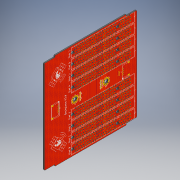
# Autodesk Inventor part: Backplane_PCB
Saved by Autodesk Inventor 2018 (Build 220112000, 112)
## iProperties
Created: 2018-10-18
Part Number: Backplane_PCB
Material: Epoxy Resin
Document SubType Name: Modeling
Designer: Bradley
Density: 1.14 g/cm^3
Appearance: Smooth - Dark Gray
Author: Bradley
Autodesk Inventor part; units mm, degrees
ref_plane "YZ Plane" through (0, 0, 0) normal (1, 0, 0) x (0, 1, 0)
ref_plane "XZ Plane" through (0, 0, 0) normal (0, 1, 0) x (-1, 0, 0)
ref_plane "XY Plane" through (0, 0, 0) normal (0, 0, 1) x (1, 0, 0)
sketch "Sketch11" plane through (0, 0, 0) normal (1, 0, 0) x (0, 1, 0)
  line L0 (-41.4, 41.6) -> (-32, 41.6)
  line L1 (-32, 41.6) -> (-32, 43)
  line L2 (-32, 43) -> (32, 43)
  line L3 (32, 43) -> (32, 41.6)
  line L4 (32, 41.6) -> (41.4, 41.6)
  line L5 (41.4, 41.6) -> (41.4, -41.6)
  line L6 (41.4, -41.6) -> (32, -41.6)
  line L7 (32, -41.6) -> (32, -43)
  line L8 (32, -43) -> (-32, -43)
  line L9 (-32, -43) -> (-32, -41.6)
  line L10 (-32, -41.6) -> (-41.4, -41.6)
  line L11 (-41.4, -41.6) -> (-41.4, 41.6)
  point P0 (0, 0)
  point P1 (0, 43)
  point P2 (-41.4, 0)
  dimension "d86" = 83.2
  dimension "d87" = 9.4
  dimension "d88" = 82.8
  dimension "d89" = 86
  constraints: 24 end point, 8 perpendicular, 5 point on line, 3 collinear, 2 midpoint, 1 horizontal, 1 horizontal alignment, 1 vertical, 1 vertical alignment
  measures "d86" distance of L4.end L5.end
  measures "d87" distance of L3.end L4.end
  measures "d88" distance between parallel lines of L11 L5
  measures "d89" distance between parallel lines of L8 L2
extrude "Extrusion3" add sketch "Sketch11" along normal mid plane 1
fillet "Fillet2" radius 0.5 12 edges at (0, -32, 43) (0, -32, 41.6) (0, -41.4, 41.6) (0, -32, -41.6) (0, -32, -43) (0, -41.4, -41.6) (0, 32, -43) (0, 32, -41.6) (0, 41.4, -41.6) (0, 32, 43) (0, 32, 41.6) (0, 41.4, 41.6)
sketch "Sketch12" plane through (0.5, 0, 0) normal (1, 0, 0) x (0, 0, -1)
  arc A0 (-41.1, 41.4) -> (-41.6, 40.9) centre (-41.1, 40.9) ccw projected
  line L0 (-41.6, 40.9) -> (-41.6, 32.5) projected
  arc A1 (-42.1, 32) -> (-41.6, 32.5) centre (-42.1, 32.5) ccw projected
  line L1 (-42.1, 32) -> (-42.5, 32) projected
  arc A2 (-42.5, 32) -> (-43, 31.5) centre (-42.5, 31.5) ccw projected
  line L2 (-43, 31.5) -> (-43, -31.5) projected
  arc A3 (-43, -31.5) -> (-42.5, -32) centre (-42.5, -31.5) ccw projected
  line L3 (-42.5, -32) -> (-42.1, -32) projected
  arc A4 (-41.6, -32.5) -> (-42.1, -32) centre (-42.1, -32.5) ccw projected
  line L4 (-41.6, -32.5) -> (-41.6, -40.9) projected
  arc A5 (-41.6, -40.9) -> (-41.1, -41.4) centre (-41.1, -40.9) ccw projected
  line L5 (-41.1, -41.4) -> (41.1, -41.4) projected
  arc A6 (41.1, -41.4) -> (41.6, -40.9) centre (41.1, -40.9) ccw projected
  line L6 (41.6, -40.9) -> (41.6, -32.5) projected
  arc A7 (42.1, -32) -> (41.6, -32.5) centre (42.1, -32.5) ccw projected
  line L7 (42.1, -32) -> (42.5, -32) projected
  arc A8 (42.5, -32) -> (43, -31.5) centre (42.5, -31.5) ccw projected
  line L8 (43, -31.5) -> (43, 31.5) projected
  arc A9 (43, 31.5) -> (42.5, 32) centre (42.5, 31.5) ccw projected
  line L9 (42.5, 32) -> (42.1, 32) projected
  arc A10 (41.6, 32.5) -> (42.1, 32) centre (42.1, 32.5) ccw projected
  line L10 (41.6, 32.5) -> (41.6, 40.9) projected
  arc A11 (41.6, 40.9) -> (41.1, 41.4) centre (41.1, 40.9) ccw projected
  line L11 (41.1, 41.4) -> (-41.1, 41.4) projected
  line L12 (-42.9956, -41.4) -> (-42.9956, 41.4) construction
  line L13 (-42.9956, 41.4) -> (42.9956, 41.4) construction
  line L14 (42.9956, 41.4) -> (42.9956, -41.4) construction
  line L15 (42.9956, -41.4) -> (-42.9956, -41.4) construction
  line L16 (-41.1, -41.4) -> (41.1, -41.4) projected
  point P0 (0, 0)
  point P1 (0, -41.4)
  point P2 (0, -41.4)
  constraints: 3 midpoint, 2 collinear, 2 other
decal "Decal3"
sketch "Sketch13" plane through (-0.5, 0, 0) normal (-1, 0, 0) x (0, 0, 1)
  arc A0 (41.6, 40.9) -> (41.1, 41.4) centre (41.1, 40.9) ccw projected
  line L0 (41.1, 41.4) -> (-41.1, 41.4) projected
  arc A1 (-41.1, 41.4) -> (-41.6, 40.9) centre (-41.1, 40.9) ccw projected
  line L1 (-41.6, 40.9) -> (-41.6, 32.5) projected
  arc A2 (-42.1, 32) -> (-41.6, 32.5) centre (-42.1, 32.5) ccw projected
  line L2 (-42.1, 32) -> (-42.5, 32) projected
  arc A3 (-42.5, 32) -> (-43, 31.5) centre (-42.5, 31.5) ccw projected
  line L3 (-43, 31.5) -> (-43, -31.5) projected
  arc A4 (-43, -31.5) -> (-42.5, -32) centre (-42.5, -31.5) ccw projected
  line L4 (-42.5, -32) -> (-42.1, -32) projected
  arc A5 (-41.6, -32.5) -> (-42.1, -32) centre (-42.1, -32.5) ccw projected
  line L5 (-41.6, -32.5) -> (-41.6, -40.9) projected
  arc A6 (-41.6, -40.9) -> (-41.1, -41.4) centre (-41.1, -40.9) ccw projected
  line L6 (-41.1, -41.4) -> (41.1, -41.4) projected
  arc A7 (41.1, -41.4) -> (41.6, -40.9) centre (41.1, -40.9) ccw projected
  line L7 (41.6, -40.9) -> (41.6, -32.5) projected
  arc A8 (42.1, -32) -> (41.6, -32.5) centre (42.1, -32.5) ccw projected
  line L8 (42.1, -32) -> (42.5, -32) projected
  arc A9 (42.5, -32) -> (43, -31.5) centre (42.5, -31.5) ccw projected
  line L9 (43, -31.5) -> (43, 31.5) projected
  arc A10 (43, 31.5) -> (42.5, 32) centre (42.5, 31.5) ccw projected
  line L10 (42.5, 32) -> (42.1, 32) projected
  arc A11 (41.6, 32.5) -> (42.1, 32) centre (42.1, 32.5) ccw projected
  line L11 (41.6, 32.5) -> (41.6, 40.9) projected
  line L12 (41.1, 41.4) -> (-41.1, 41.4) projected
  line L13 (42.9956, 41.4) -> (42.9956, -41.4) construction
  line L14 (42.9956, -41.4) -> (-42.9956, -41.4) construction
  line L15 (-42.9956, -41.4) -> (-42.9956, 41.4) construction
  line L16 (-42.9956, 41.4) -> (42.9956, 41.4) construction
  line L17 (-41.1, -41.4) -> (41.1, -41.4) projected
  point P0 (0, 0)
  point P1 (0, -41.4)
  point P2 (0, -41.4)
  constraints: 3 midpoint, 2 collinear, 2 other
decal "Decal4"
sketch "Sketch14" plane through (0.5, 0, 0) normal (1, 0, 0) x (0, 0, -1)
  point P0 (0, 0)
  point P1 (0, -14)
  point P2 (0, 14)
  constraints: 2 other
hole "Hole7" at (0.5, -14, 0) at (0.5, 14, 0) direction (-1, 0, 0) diameter 3.3 end through all
sketch "Sketch15" plane through (0.5, 0, 0) normal (1, 0, 0) x (0, 0, -1)
  point P0 (0, 0)
  point P1 (37.5, 24)
  point P2 (37.5, -16.15)
  point P3 (-37.5, 24)
  point P4 (-37.5, -16.15)
  point P5 (28.5, 24)
  point P6 (28.5, -16.15)
  point P7 (19.5, 24)
  point P8 (19.5, -16.15)
  point P9 (10.5, 24)
  point P10 (10.5, -16.15)
  point P11 (-10.5, 24)
  point P12 (-10.5, -16.15)
  point P13 (-19.5, 24)
  point P14 (-19.5, -16.15)
  point P15 (-28.5, 24)
  point P16 (-28.5, -16.15)
  constraints: 16 other
hole "Hole8" at (0.5, 24, -37.5) at (0.5, -16.15, -37.5) at (0.5, 24, 37.5) at (0.5, -16.15, 37.5) at (0.5, 24, -28.5) at (0.5, -16.15, -28.5) at (0.5, 24, -19.5) at (0.5, -16.15, -19.5) at (0.5, 24, -10.5) at (0.5, -16.15, -10.5) at (0.5, 24, 10.5) at (0.5, -16.15, 10.5) at (0.5, 24, 19.5) at (0.5, -16.15, 19.5) at (0.5, 24, 28.5) at (0.5, -16.15, 28.5) direction (-1, 0, 0) diameter 2.35 end through all
sketch "Sketch16" plane through (0.5, 0, 0) normal (1, 0, 0) x (0, 0, -1)
  point P0 (0, 0)
  point P1 (40.75, 0.65)
  point P2 (-29.75, -6.35)
  point P3 (-31.75, -7.35)
  point P4 (-25.25, -7.35)
  point P5 (-27.25, -8.35)
  point P6 (-29.75, -8.35)
  point P7 (-31.75, -9.35)
  point P8 (-25.25, -9.35)
  point P9 (-27.25, -10.35)
  point P10 (-29.75, -10.35)
  point P11 (-31.75, -11.35)
  point P12 (-25.25, -11.35)
  point P13 (-27.25, -12.35)
  point P14 (-29.75, -12.35)
  point P15 (-31.75, -13.35)
  point P16 (-25.25, -13.35)
  point P17 (-27.25, -14.35)
  point P18 (36.25, 25.65)
  point P19 (34.25, 26.65)
  point P20 (40.75, 26.65)
  point P21 (38.75, 25.65)
  point P22 (36.25, 27.65)
  point P23 (34.25, 28.65)
  point P24 (40.75, 28.65)
  point P25 (38.75, 27.65)
  point P26 (36.25, 29.65)
  point P27 (34.25, 30.65)
  point P28 (40.75, 30.65)
  point P29 (38.75, 29.65)
  point P30 (36.25, 31.65)
  point P31 (34.25, 32.65)
  point P32 (40.75, 32.65)
  point P33 (38.75, 31.65)
  point P34 (36.25, 33.65)
  point P35 (34.25, 34.65)
  point P36 (40.75, 34.65)
  point P37 (38.75, 33.65)
  point P38 (36.25, 35.65)
  point P39 (38.75, 35.65)
  point P40 (34.25, 22.65)
  point P41 (40.75, 22.65)
  point P42 (38.75, 21.65)
  point P43 (36.25, 21.65)
  point P44 (34.25, 20.65)
  point P45 (40.75, 20.65)
  point P46 (38.75, 19.65)
  point P47 (36.25, 19.65)
  point P48 (34.25, 18.65)
  point P49 (40.75, 18.65)
  point P50 (38.75, 17.65)
  point P51 (36.25, 17.65)
  point P52 (34.25, 16.65)
  point P53 (40.75, 16.65)
  point P54 (38.75, 15.65)
  point P55 (36.25, 15.65)
  point P56 (34.25, 14.65)
  point P57 (40.75, 14.65)
  point P58 (38.75, 13.65)
  point P59 (36.25, 13.65)
  point P60 (34.25, 12.65)
  point P61 (40.75, 12.65)
  point P62 (38.75, 11.65)
  point P63 (36.25, 11.65)
  point P64 (34.25, 10.65)
  point P65 (40.75, 10.65)
  point P66 (38.75, 9.65)
  point P67 (36.25, 9.65)
  point P68 (34.25, 8.65)
  point P69 (40.75, 8.65)
  point P70 (38.75, 7.65)
  point P71 (36.25, 7.65)
  point P72 (34.25, 6.65)
  point P73 (40.75, 6.65)
  point P74 (38.75, 5.65)
  point P75 (36.25, 5.65)
  point P76 (34.25, 4.65)
  point P77 (40.75, 4.65)
  point P78 (38.75, 3.65)
  point P79 (36.25, 3.65)
  point P80 (34.25, 2.65)
  point P81 (40.75, 2.65)
  point P82 (38.75, 1.65)
  point P83 (36.25, 1.65)
  point P84 (34.25, 0.65)
  point P85 (-34.25, -1.35)
  point P86 (38.75, -0.35)
  point P87 (36.25, -0.35)
  point P88 (34.25, -1.35)
  point P89 (40.75, -1.35)
  point P90 (38.75, -2.35)
  point P91 (36.25, -2.35)
  point P92 (34.25, -3.35)
  point P93 (40.75, -3.35)
  point P94 (38.75, -4.35)
  point P95 (36.25, -4.35)
  point P96 (34.25, -5.35)
  point P97 (40.75, -5.35)
  point P98 (38.75, -6.35)
  point P99 (36.25, -6.35)
  point P100 (34.25, -7.35)
  point P101 (40.75, -7.35)
  point P102 (38.75, -8.35)
  point P103 (36.25, -8.35)
  point P104 (34.25, -9.35)
  point P105 (40.75, -9.35)
  point P106 (38.75, -10.35)
  point P107 (36.25, -10.35)
  point P108 (34.25, -11.35)
  point P109 (40.75, -11.35)
  point P110 (38.75, -12.35)
  point P111 (36.25, -12.35)
  point P112 (34.25, -13.35)
  point P113 (40.75, -13.35)
  point P114 (38.75, -14.35)
  point P115 (36.25, -14.35)
  point P116 (-38.75, 25.65)
  point P117 (-40.75, 26.65)
  point P118 (-34.25, 26.65)
  point P119 (-36.25, 25.65)
  point P120 (-38.75, 27.65)
  point P121 (-40.75, 28.65)
  point P122 (-34.25, 28.65)
  point P123 (-36.25, 27.65)
  point P124 (-38.75, 29.65)
  point P125 (-40.75, 30.65)
  point P126 (-34.25, 30.65)
  point P127 (-36.25, 29.65)
  point P128 (-38.75, 31.65)
  point P129 (-40.75, 32.65)
  point P130 (-34.25, 32.65)
  point P131 (-36.25, 31.65)
  point P132 (-38.75, 33.65)
  point P133 (-40.75, 34.65)
  point P134 (-34.25, 34.65)
  point P135 (-36.25, 33.65)
  point P136 (-38.75, 35.65)
  point P137 (-36.25, 35.65)
  point P138 (-40.75, 22.65)
  point P139 (-34.25, 22.65)
  point P140 (-36.25, 21.65)
  point P141 (-38.75, 21.65)
  point P142 (-40.75, 20.65)
  point P143 (-34.25, 20.65)
  point P144 (-36.25, 19.65)
  point P145 (-38.75, 19.65)
  point P146 (-40.75, 18.65)
  point P147 (-34.25, 18.65)
  point P148 (-36.25, 17.65)
  point P149 (-38.75, 17.65)
  point P150 (-40.75, 16.65)
  point P151 (-34.25, 16.65)
  point P152 (-36.25, 15.65)
  point P153 (-38.75, 15.65)
  point P154 (-40.75, 14.65)
  point P155 (-34.25, 14.65)
  point P156 (-36.25, 13.65)
  point P157 (-38.75, 13.65)
  point P158 (-40.75, 12.65)
  point P159 (-34.25, 12.65)
  point P160 (-36.25, 11.65)
  point P161 (-38.75, 11.65)
  point P162 (-40.75, 10.65)
  point P163 (-34.25, 10.65)
  point P164 (-36.25, 9.65)
  point P165 (-38.75, 9.65)
  point P166 (-40.75, 8.65)
  point P167 (-34.25, 8.65)
  point P168 (-36.25, 7.65)
  point P169 (-38.75, 7.65)
  point P170 (-40.75, 6.65)
  point P171 (-34.25, 6.65)
  point P172 (-36.25, 5.65)
  point P173 (-38.75, 5.65)
  point P174 (-40.75, 4.65)
  point P175 (-34.25, 4.65)
  point P176 (-36.25, 3.65)
  point P177 (-38.75, 3.65)
  point P178 (-40.75, 2.65)
  point P179 (-34.25, 2.65)
  point P180 (-36.25, 1.65)
  point P181 (-38.75, 1.65)
  point P182 (-40.75, 0.65)
  point P183 (-34.25, 0.65)
  point P184 (-36.25, -0.35)
  point P185 (-38.75, -0.35)
  point P186 (-40.75, -1.35)
  point P187 (-29.75, -14.35)
  point P188 (-36.25, -2.35)
  point P189 (-38.75, -2.35)
  point P190 (-40.75, -3.35)
  point P191 (-34.25, -3.35)
  point P192 (-36.25, -4.35)
  point P193 (-38.75, -4.35)
  point P194 (-40.75, -5.35)
  point P195 (-34.25, -5.35)
  point P196 (-36.25, -6.35)
  point P197 (-38.75, -6.35)
  point P198 (-40.75, -7.35)
  point P199 (-34.25, -7.35)
  constraints: 784 other
hole "Hole9" at (0.5, 0.65, -40.75) at (0.5, -6.35, 29.75) at (0.5, -7.35, 31.75) at (0.5, -7.35, 25.25) at (0.5, -8.35, 27.25) at (0.5, -8.35, 29.75) at (0.5, -9.35, 31.75) at (0.5, -9.35, 25.25) at (0.5, -10.35, 27.25) at (0.5, -10.35, 29.75) at (0.5, -11.35, 31.75) at (0.5, -11.35, 25.25) at (0.5, -12.35, 27.25) at (0.5, -12.35, 29.75) at (0.5, -13.35, 31.75) at (0.5, -13.35, 25.25) at (0.5, -14.35, 27.25) at (0.5, 25.65, -36.25) at (0.5, 26.65, -34.25) at (0.5, 26.65, -40.75) at (0.5, 25.65, -38.75) at (0.5, 27.65, -36.25) at (0.5, 28.65, -34.25) at (0.5, 28.65, -40.75) at (0.5, 27.65, -38.75) at (0.5, 29.65, -36.25) at (0.5, 30.65, -34.25) at (0.5, 30.65, -40.75) at (0.5, 29.65, -38.75) at (0.5, 31.65, -36.25) at (0.5, 32.65, -34.25) at (0.5, 32.65, -40.75) at (0.5, 31.65, -38.75) at (0.5, 33.65, -36.25) at (0.5, 34.65, -34.25) at (0.5, 34.65, -40.75) at (0.5, 33.65, -38.75) at (0.5, 35.65, -36.25) at (0.5, 35.65, -38.75) at (0.5, 22.65, -34.25) at (0.5, 22.65, -40.75) at (0.5, 21.65, -38.75) at (0.5, 21.65, -36.25) at (0.5, 20.65, -34.25) at (0.5, 20.65, -40.75) at (0.5, 19.65, -38.75) at (0.5, 19.65, -36.25) at (0.5, 18.65, -34.25) at (0.5, 18.65, -40.75) at (0.5, 17.65, -38.75) direction (-1, 0, 0) diameter 0.7 end through all and at (0.5, 17.65, -36.25) (0.5, 16.65, -34.25) (0.5, 16.65, -40.75) (0.5, 15.65, -38.75) (0.5, 15.65, -36.25) (0.5, 14.65, -34.25) (0.5, 14.65, -40.75) (0.5, 13.65, -38.75) (0.5, 13.65, -36.25) (0.5, 12.65, -34.25) (0.5, 12.65, -40.75) (0.5, 11.65, -38.75) (0.5, 11.65, -36.25) (0.5, 10.65, -34.25) (0.5, 10.65, -40.75) (0.5, 9.65, -38.75) (0.5, 9.65, -36.25) (0.5, 8.65, -34.25) (0.5, 8.65, -40.75) (0.5, 7.65, -38.75) (0.5, 7.65, -36.25) (0.5, 6.65, -34.25) (0.5, 6.65, -40.75) (0.5, 5.65, -38.75) (0.5, 5.65, -36.25) (0.5, 4.65, -34.25) (0.5, 4.65, -40.75) (0.5, 3.65, -38.75) (0.5, 3.65, -36.25) (0.5, 2.65, -34.25) (0.5, 2.65, -40.75) (0.5, 1.65, -38.75) (0.5, 1.65, -36.25) (0.5, 0.65, -34.25) (0.5, -1.35, 34.25) (0.5, -0.35, -38.75) (0.5, -0.35, -36.25) (0.5, -1.35, -34.25) (0.5, -1.35, -40.75) (0.5, -2.35, -38.75) (0.5, -2.35, -36.25) (0.5, -3.35, -34.25) (0.5, -3.35, -40.75) (0.5, -4.35, -38.75) (0.5, -4.35, -36.25) (0.5, -5.35, -34.25) (0.5, -5.35, -40.75) (0.5, -6.35, -38.75) (0.5, -6.35, -36.25) (0.5, -7.35, -34.25) (0.5, -7.35, -40.75) (0.5, -8.35, -38.75) (0.5, -8.35, -36.25) (0.5, -9.35, -34.25) (0.5, -9.35, -40.75) (0.5, -10.35, -38.75) (0.5, -10.35, -36.25) (0.5, -11.35, -34.25) (0.5, -11.35, -40.75) (0.5, -12.35, -38.75) (0.5, -12.35, -36.25) (0.5, -13.35, -34.25) (0.5, -13.35, -40.75) (0.5, -14.35, -38.75) (0.5, -14.35, -36.25) (0.5, 25.65, 38.75) (0.5, 26.65, 40.75) (0.5, 26.65, 34.25) (0.5, 25.65, 36.25) (0.5, 27.65, 38.75) (0.5, 28.65, 40.75) (0.5, 28.65, 34.25) (0.5, 27.65, 36.25) (0.5, 29.65, 38.75) (0.5, 30.65, 40.75) (0.5, 30.65, 34.25) (0.5, 29.65, 36.25) (0.5, 31.65, 38.75) (0.5, 32.65, 40.75) (0.5, 32.65, 34.25) (0.5, 31.65, 36.25) (0.5, 33.65, 38.75) (0.5, 34.65, 40.75) (0.5, 34.65, 34.25) (0.5, 33.65, 36.25) (0.5, 35.65, 38.75) (0.5, 35.65, 36.25) (0.5, 22.65, 40.75) (0.5, 22.65, 34.25) (0.5, 21.65, 36.25) (0.5, 21.65, 38.75) (0.5, 20.65, 40.75) (0.5, 20.65, 34.25) (0.5, 19.65, 36.25) (0.5, 19.65, 38.75) (0.5, 18.65, 40.75) (0.5, 18.65, 34.25) (0.5, 17.65, 36.25) (0.5, 17.65, 38.75) (0.5, 16.65, 40.75) (0.5, 16.65, 34.25) (0.5, 15.65, 36.25) (0.5, 15.65, 38.75) (0.5, 14.65, 40.75) (0.5, 14.65, 34.25) (0.5, 13.65, 36.25) (0.5, 13.65, 38.75) (0.5, 12.65, 40.75) (0.5, 12.65, 34.25) (0.5, 11.65, 36.25) (0.5, 11.65, 38.75) (0.5, 10.65, 40.75) (0.5, 10.65, 34.25) (0.5, 9.65, 36.25) (0.5, 9.65, 38.75) (0.5, 8.65, 40.75) (0.5, 8.65, 34.25) (0.5, 7.65, 36.25) (0.5, 7.65, 38.75) (0.5, 6.65, 40.75) (0.5, 6.65, 34.25) (0.5, 5.65, 36.25) (0.5, 5.65, 38.75) (0.5, 4.65, 40.75) (0.5, 4.65, 34.25) (0.5, 3.65, 36.25) (0.5, 3.65, 38.75) (0.5, 2.65, 40.75) (0.5, 2.65, 34.25) (0.5, 1.65, 36.25) (0.5, 1.65, 38.75) (0.5, 0.65, 40.75) (0.5, 0.65, 34.25) (0.5, -0.35, 36.25) (0.5, -0.35, 38.75) (0.5, -1.35, 40.75) (0.5, -14.35, 29.75) (0.5, -2.35, 36.25) (0.5, -2.35, 38.75) (0.5, -3.35, 40.75) (0.5, -3.35, 34.25) (0.5, -4.35, 36.25) (0.5, -4.35, 38.75) (0.5, -5.35, 40.75) (0.5, -5.35, 34.25) (0.5, -6.35, 36.25) (0.5, -6.35, 38.75) (0.5, -7.35, 40.75) (0.5, -7.35, 34.25) (0.5, -8.35, 36.25) (0.5, -8.35, 38.75) (0.5, -9.35, 40.75) (0.5, -9.35, 34.25) (0.5, -10.35, 36.25) (0.5, -10.35, 38.75) (0.5, -11.35, 40.75) (0.5, -11.35, 34.25) (0.5, -12.35, 36.25) (0.5, -12.35, 38.75) (0.5, -13.35, 40.75) (0.5, -13.35, 34.25) (0.5, -14.35, 36.25) (0.5, -14.35, 38.75) (0.5, 25.65, -27.25) (0.5, 26.65, -25.25) (0.5, 26.65, -31.75) (0.5, 25.65, -29.75) (0.5, 27.65, -27.25) (0.5, 28.65, -25.25) (0.5, 28.65, -31.75) (0.5, 27.65, -29.75) (0.5, 29.65, -27.25) (0.5, 30.65, -25.25) (0.5, 30.65, -31.75) (0.5, 29.65, -29.75) (0.5, 31.65, -27.25) (0.5, 32.65, -25.25) (0.5, 32.65, -31.75) (0.5, 31.65, -29.75) (0.5, 33.65, -27.25) (0.5, 34.65, -25.25) (0.5, 34.65, -31.75) (0.5, 33.65, -29.75) (0.5, 35.65, -27.25) (0.5, 35.65, -29.75) (0.5, 22.65, -25.25) (0.5, 22.65, -31.75) (0.5, 21.65, -29.75) (0.5, 21.65, -27.25) (0.5, 20.65, -25.25) (0.5, 20.65, -31.75) (0.5, 19.65, -29.75) (0.5, 19.65, -27.25) (0.5, 18.65, -25.25) (0.5, 18.65, -31.75) (0.5, 17.65, -29.75) (0.5, 17.65, -27.25) (0.5, 16.65, -25.25) (0.5, 16.65, -31.75) (0.5, 15.65, -29.75) (0.5, 15.65, -27.25) (0.5, 14.65, -25.25) (0.5, 14.65, -31.75) (0.5, 13.65, -29.75) (0.5, 13.65, -27.25) (0.5, 12.65, -25.25) (0.5, 12.65, -31.75) (0.5, 11.65, -29.75) (0.5, 11.65, -27.25) (0.5, 10.65, -25.25) (0.5, 10.65, -31.75) (0.5, 9.65, -29.75) (0.5, 9.65, -27.25) (0.5, 8.65, -25.25) (0.5, 8.65, -31.75) (0.5, 7.65, -29.75) (0.5, 7.65, -27.25) (0.5, 6.65, -25.25) (0.5, 6.65, -31.75) (0.5, 5.65, -29.75) (0.5, 5.65, -27.25) (0.5, 4.65, -25.25) (0.5, 4.65, -31.75) (0.5, 3.65, -29.75) (0.5, 3.65, -27.25) (0.5, 2.65, -25.25) (0.5, 2.65, -31.75) (0.5, 1.65, -29.75) (0.5, 1.65, -27.25) (0.5, 0.65, -25.25) (0.5, 0.65, -31.75) (0.5, -0.35, -29.75) (0.5, -0.35, -27.25) (0.5, -1.35, -25.25) (0.5, -1.35, -31.75) (0.5, -2.35, -29.75) (0.5, -2.35, -27.25) (0.5, -3.35, -25.25) (0.5, -3.35, -31.75) (0.5, -4.35, -29.75) (0.5, -4.35, -27.25) (0.5, -5.35, -25.25) (0.5, -5.35, -31.75) (0.5, -6.35, -29.75) (0.5, -6.35, -27.25) (0.5, -7.35, -25.25) (0.5, -7.35, -31.75) (0.5, -8.35, -29.75) (0.5, -8.35, -27.25) (0.5, -9.35, -25.25) (0.5, -9.35, -31.75) (0.5, -10.35, -29.75) (0.5, -10.35, -27.25) (0.5, -11.35, -25.25) (0.5, -11.35, -31.75) (0.5, -12.35, -29.75) (0.5, -12.35, -27.25) (0.5, -13.35, -25.25) (0.5, -13.35, -31.75) (0.5, -14.35, -29.75) (0.5, -14.35, -27.25) (0.5, 25.65, -18.25) (0.5, 26.65, -16.25) (0.5, 26.65, -22.75) (0.5, 25.65, -20.75) (0.5, 27.65, -18.25) (0.5, 28.65, -16.25) (0.5, 28.65, -22.75) (0.5, 27.65, -20.75) (0.5, 29.65, -18.25) (0.5, 30.65, -16.25) (0.5, 30.65, -22.75) (0.5, 29.65, -20.75) (0.5, 31.65, -18.25) (0.5, 32.65, -16.25) (0.5, 32.65, -22.75) (0.5, 31.65, -20.75) (0.5, 33.65, -18.25) (0.5, 34.65, -16.25) (0.5, 34.65, -22.75) (0.5, 33.65, -20.75) (0.5, 35.65, -18.25) (0.5, 35.65, -20.75) (0.5, 22.65, -16.25) (0.5, 22.65, -22.75) (0.5, 21.65, -20.75) (0.5, 21.65, -18.25) (0.5, 20.65, -16.25) (0.5, 20.65, -22.75) (0.5, 19.65, -20.75) (0.5, 19.65, -18.25) (0.5, 18.65, -16.25) (0.5, 18.65, -22.75) (0.5, 17.65, -20.75) (0.5, 17.65, -18.25) (0.5, 16.65, -16.25) (0.5, 16.65, -22.75) (0.5, 15.65, -20.75) (0.5, 15.65, -18.25) (0.5, 14.65, -16.25) (0.5, 14.65, -22.75) (0.5, 13.65, -20.75) (0.5, 13.65, -18.25) (0.5, 12.65, -16.25) (0.5, 12.65, -22.75) (0.5, 11.65, -20.75) (0.5, 11.65, -18.25) (0.5, 10.65, -16.25) (0.5, 10.65, -22.75) (0.5, 9.65, -20.75) (0.5, 9.65, -18.25) (0.5, 8.65, -16.25) (0.5, 8.65, -22.75) (0.5, 7.65, -20.75) (0.5, 7.65, -18.25) (0.5, 6.65, -16.25) (0.5, 6.65, -22.75) (0.5, 5.65, -20.75) (0.5, 5.65, -18.25) (0.5, 4.65, -16.25) (0.5, 4.65, -22.75) (0.5, 3.65, -20.75) (0.5, 3.65, -18.25) (0.5, 2.65, -16.25) (0.5, 2.65, -22.75) (0.5, 1.65, -20.75) (0.5, 1.65, -18.25) (0.5, 0.65, -16.25) (0.5, 0.65, -22.75) (0.5, -0.35, -20.75) (0.5, -0.35, -18.25) (0.5, -1.35, -16.25) (0.5, -1.35, -22.75) (0.5, -2.35, -20.75) (0.5, -2.35, -18.25) (0.5, -3.35, -16.25) (0.5, -3.35, -22.75) (0.5, -4.35, -20.75) (0.5, -4.35, -18.25) (0.5, -5.35, -16.25) (0.5, -5.35, -22.75) (0.5, -6.35, -20.75) (0.5, -6.35, -18.25) (0.5, -7.35, -16.25) (0.5, -7.35, -22.75) (0.5, -8.35, -20.75) (0.5, -8.35, -18.25) (0.5, -9.35, -16.25) (0.5, -9.35, -22.75) (0.5, -10.35, -20.75) (0.5, -10.35, -18.25) (0.5, -11.35, -16.25) (0.5, -11.35, -22.75) (0.5, -12.35, -20.75) (0.5, -12.35, -18.25) (0.5, -13.35, -16.25) (0.5, -13.35, -22.75) (0.5, -14.35, -20.75) (0.5, -14.35, -18.25) (0.5, 25.65, -9.25) (0.5, 26.65, -7.25) (0.5, 26.65, -13.75) (0.5, 25.65, -11.75) (0.5, 27.65, -9.25) (0.5, 28.65, -7.25) (0.5, 28.65, -13.75) (0.5, 27.65, -11.75) (0.5, 29.65, -9.25) (0.5, 30.65, -7.25) (0.5, 30.65, -13.75) (0.5, 29.65, -11.75) (0.5, 31.65, -9.25) (0.5, 32.65, -7.25) (0.5, 32.65, -13.75) (0.5, 31.65, -11.75) (0.5, 33.65, -9.25) (0.5, 34.65, -7.25) (0.5, 34.65, -13.75) (0.5, 33.65, -11.75) (0.5, 35.65, -9.25) (0.5, 35.65, -11.75) (0.5, 22.65, -7.25) (0.5, 22.65, -13.75) (0.5, 21.65, -11.75) (0.5, 21.65, -9.25) (0.5, 20.65, -7.25) (0.5, 20.65, -13.75) (0.5, 19.65, -11.75) (0.5, 19.65, -9.25) (0.5, 18.65, -7.25) (0.5, 18.65, -13.75) (0.5, 17.65, -11.75) (0.5, 17.65, -9.25) (0.5, 16.65, -7.25) (0.5, 16.65, -13.75) (0.5, 15.65, -11.75) (0.5, 15.65, -9.25) (0.5, 14.65, -7.25) (0.5, 14.65, -13.75) (0.5, 13.65, -11.75) (0.5, 13.65, -9.25) (0.5, 12.65, -7.25) (0.5, 12.65, -13.75) (0.5, 11.65, -11.75) (0.5, 11.65, -9.25) (0.5, 10.65, -7.25) (0.5, 10.65, -13.75) (0.5, 9.65, -11.75) (0.5, 9.65, -9.25) (0.5, 8.65, -7.25) (0.5, 8.65, -13.75) (0.5, 7.65, -11.75) (0.5, 7.65, -9.25) (0.5, 6.65, -7.25) (0.5, 6.65, -13.75) (0.5, 5.65, -11.75) (0.5, 5.65, -9.25) (0.5, 4.65, -7.25) (0.5, 4.65, -13.75) (0.5, 3.65, -11.75) (0.5, 3.65, -9.25) (0.5, 2.65, -7.25) (0.5, 2.65, -13.75) (0.5, 1.65, -11.75) (0.5, 1.65, -9.25) (0.5, 0.65, -7.25) (0.5, 0.65, -13.75) (0.5, -0.35, -11.75) (0.5, -0.35, -9.25) (0.5, -1.35, -7.25) (0.5, -1.35, -13.75) (0.5, -2.35, -11.75) (0.5, -2.35, -9.25) (0.5, -3.35, -7.25) (0.5, -3.35, -13.75) (0.5, -4.35, -11.75) (0.5, -4.35, -9.25) (0.5, -5.35, -7.25) (0.5, -5.35, -13.75) (0.5, -6.35, -11.75) (0.5, -6.35, -9.25) (0.5, -7.35, -7.25) (0.5, -7.35, -13.75) (0.5, -8.35, -11.75) (0.5, -8.35, -9.25) (0.5, -9.35, -7.25) (0.5, -9.35, -13.75) (0.5, -10.35, -11.75) (0.5, -10.35, -9.25) (0.5, -11.35, -7.25) (0.5, -11.35, -13.75) (0.5, -12.35, -11.75) (0.5, -12.35, -9.25) (0.5, -13.35, -7.25) (0.5, -13.35, -13.75) (0.5, -14.35, -11.75) (0.5, -14.35, -9.25) (0.5, 25.65, 11.75) (0.5, 26.65, 13.75) (0.5, 26.65, 7.25) (0.5, 25.65, 9.25) (0.5, 27.65, 11.75) (0.5, 28.65, 13.75) (0.5, 28.65, 7.25) (0.5, 27.65, 9.25) (0.5, 29.65, 11.75) (0.5, 30.65, 13.75) (0.5, 30.65, 7.25) (0.5, 29.65, 9.25) (0.5, 31.65, 11.75) (0.5, 32.65, 13.75) (0.5, 32.65, 7.25) (0.5, 31.65, 9.25) (0.5, 33.65, 11.75) (0.5, 34.65, 13.75) (0.5, 34.65, 7.25) (0.5, 33.65, 9.25) (0.5, 35.65, 11.75) (0.5, 35.65, 9.25) (0.5, 22.65, 13.75) (0.5, 22.65, 7.25) (0.5, 21.65, 9.25) (0.5, 21.65, 11.75) (0.5, 20.65, 13.75) (0.5, 20.65, 7.25) (0.5, 19.65, 9.25) (0.5, 19.65, 11.75) (0.5, 18.65, 13.75) (0.5, 18.65, 7.25) (0.5, 17.65, 9.25) (0.5, 17.65, 11.75) (0.5, 16.65, 13.75) (0.5, 16.65, 7.25) (0.5, 15.65, 9.25) (0.5, 15.65, 11.75) (0.5, 14.65, 13.75) (0.5, 14.65, 7.25) (0.5, 13.65, 9.25) (0.5, 13.65, 11.75) (0.5, 12.65, 13.75) (0.5, 12.65, 7.25) (0.5, 11.65, 9.25) (0.5, 11.65, 11.75) (0.5, 10.65, 13.75) (0.5, 10.65, 7.25) (0.5, 9.65, 9.25) (0.5, 9.65, 11.75) (0.5, 8.65, 13.75) (0.5, 8.65, 7.25) (0.5, 7.65, 9.25) (0.5, 7.65, 11.75) (0.5, 6.65, 13.75) (0.5, 6.65, 7.25) (0.5, 5.65, 9.25) (0.5, 5.65, 11.75) (0.5, 4.65, 13.75) (0.5, 4.65, 7.25) (0.5, 3.65, 9.25) (0.5, 3.65, 11.75) (0.5, 2.65, 13.75) (0.5, 2.65, 7.25) (0.5, 1.65, 9.25) (0.5, 1.65, 11.75) (0.5, 0.65, 13.75) (0.5, 0.65, 7.25) (0.5, -0.35, 9.25) (0.5, -0.35, 11.75) (0.5, -1.35, 13.75) (0.5, -1.35, 7.25) (0.5, -2.35, 9.25) (0.5, -2.35, 11.75) (0.5, -3.35, 13.75) (0.5, -3.35, 7.25) (0.5, -4.35, 9.25) (0.5, -4.35, 11.75) (0.5, -5.35, 13.75) (0.5, -5.35, 7.25) (0.5, -6.35, 9.25) (0.5, -6.35, 11.75) (0.5, -7.35, 13.75) (0.5, -7.35, 7.25) (0.5, -8.35, 9.25) (0.5, -8.35, 11.75) (0.5, -9.35, 13.75) (0.5, -9.35, 7.25) (0.5, -10.35, 9.25) (0.5, -10.35, 11.75) (0.5, -11.35, 13.75) (0.5, -11.35, 7.25) (0.5, -12.35, 9.25) (0.5, -12.35, 11.75) (0.5, -13.35, 13.75) (0.5, -13.35, 7.25) (0.5, -14.35, 9.25) (0.5, -14.35, 11.75) (0.5, 25.65, 20.75) (0.5, 26.65, 22.75) (0.5, 26.65, 16.25) (0.5, 25.65, 18.25) (0.5, 27.65, 20.75) (0.5, 28.65, 22.75) (0.5, 28.65, 16.25) (0.5, 27.65, 18.25) (0.5, 29.65, 20.75) (0.5, 30.65, 22.75) (0.5, 30.65, 16.25) (0.5, 29.65, 18.25) (0.5, 31.65, 20.75) (0.5, 32.65, 22.75) (0.5, 32.65, 16.25) (0.5, 31.65, 18.25) (0.5, 33.65, 20.75) (0.5, 34.65, 22.75) (0.5, 34.65, 16.25) (0.5, 33.65, 18.25) (0.5, 35.65, 20.75) (0.5, 35.65, 18.25) (0.5, 22.65, 22.75) (0.5, 22.65, 16.25) (0.5, 21.65, 18.25) (0.5, 21.65, 20.75) (0.5, 20.65, 22.75) (0.5, 20.65, 16.25) (0.5, 19.65, 18.25) (0.5, 19.65, 20.75) (0.5, 18.65, 22.75) (0.5, 18.65, 16.25) (0.5, 17.65, 18.25) (0.5, 17.65, 20.75) (0.5, 16.65, 22.75) (0.5, 16.65, 16.25) (0.5, 15.65, 18.25) (0.5, 15.65, 20.75) (0.5, 14.65, 22.75) (0.5, 14.65, 16.25) (0.5, 13.65, 18.25) (0.5, 13.65, 20.75) (0.5, 12.65, 22.75) (0.5, 12.65, 16.25) (0.5, 11.65, 18.25) (0.5, 11.65, 20.75) (0.5, 10.65, 22.75) (0.5, 10.65, 16.25) (0.5, 9.65, 18.25) (0.5, 9.65, 20.75) (0.5, 8.65, 22.75) (0.5, 8.65, 16.25) (0.5, 7.65, 18.25) (0.5, 7.65, 20.75) (0.5, 6.65, 22.75) (0.5, 6.65, 16.25) (0.5, 5.65, 18.25) (0.5, 5.65, 20.75) (0.5, 4.65, 22.75) (0.5, 4.65, 16.25) (0.5, 3.65, 18.25) (0.5, 3.65, 20.75) (0.5, 2.65, 22.75) (0.5, 2.65, 16.25) (0.5, 1.65, 18.25) (0.5, 1.65, 20.75) (0.5, 0.65, 22.75) (0.5, 0.65, 16.25) (0.5, -0.35, 18.25) (0.5, -0.35, 20.75) (0.5, -1.35, 22.75) (0.5, -1.35, 16.25) (0.5, -2.35, 18.25) (0.5, -2.35, 20.75) (0.5, -3.35, 22.75) (0.5, -3.35, 16.25) (0.5, -4.35, 18.25) (0.5, -4.35, 20.75) (0.5, -5.35, 22.75) (0.5, -5.35, 16.25) (0.5, -6.35, 18.25) (0.5, -6.35, 20.75) (0.5, -7.35, 22.75) (0.5, -7.35, 16.25) (0.5, -8.35, 18.25) (0.5, -8.35, 20.75) (0.5, -9.35, 22.75) (0.5, -9.35, 16.25) (0.5, -10.35, 18.25) (0.5, -10.35, 20.75) (0.5, -11.35, 22.75) (0.5, -11.35, 16.25) (0.5, -12.35, 18.25) (0.5, -12.35, 20.75) (0.5, -13.35, 22.75) (0.5, -13.35, 16.25) (0.5, -14.35, 18.25) (0.5, -14.35, 20.75) (0.5, 25.65, 29.75) (0.5, 26.65, 31.75) (0.5, 26.65, 25.25) (0.5, 25.65, 27.25) (0.5, 27.65, 29.75) (0.5, 28.65, 31.75) (0.5, 28.65, 25.25) (0.5, 27.65, 27.25) (0.5, 29.65, 29.75) (0.5, 30.65, 31.75) (0.5, 30.65, 25.25) (0.5, 29.65, 27.25) (0.5, 31.65, 29.75) (0.5, 32.65, 31.75) (0.5, 32.65, 25.25) (0.5, 31.65, 27.25) (0.5, 33.65, 29.75) (0.5, 34.65, 31.75) (0.5, 34.65, 25.25) (0.5, 33.65, 27.25) (0.5, 35.65, 29.75) (0.5, 35.65, 27.25) (0.5, 22.65, 31.75) (0.5, 22.65, 25.25) (0.5, 21.65, 27.25) (0.5, 21.65, 29.75) (0.5, 20.65, 31.75) (0.5, 20.65, 25.25) (0.5, 19.65, 27.25) (0.5, 19.65, 29.75) (0.5, 18.65, 31.75) (0.5, 18.65, 25.25) (0.5, 17.65, 27.25) (0.5, 17.65, 29.75) (0.5, 16.65, 31.75) (0.5, 16.65, 25.25) (0.5, 15.65, 27.25) (0.5, 15.65, 29.75) (0.5, 14.65, 31.75) (0.5, 14.65, 25.25) (0.5, 13.65, 27.25) (0.5, 13.65, 29.75) (0.5, 12.65, 31.75) (0.5, 12.65, 25.25) (0.5, 11.65, 27.25) (0.5, 11.65, 29.75) (0.5, 10.65, 31.75) (0.5, 10.65, 25.25) (0.5, 9.65, 27.25) (0.5, 9.65, 29.75) (0.5, 8.65, 31.75) (0.5, 8.65, 25.25) (0.5, 7.65, 27.25) (0.5, 7.65, 29.75) (0.5, 6.65, 31.75) (0.5, 6.65, 25.25) (0.5, 5.65, 27.25) (0.5, 5.65, 29.75) (0.5, 4.65, 31.75) (0.5, 4.65, 25.25) (0.5, 3.65, 27.25) (0.5, 3.65, 29.75) (0.5, 2.65, 31.75) (0.5, 2.65, 25.25) (0.5, 1.65, 27.25) (0.5, 1.65, 29.75) (0.5, 0.65, 31.75) (0.5, 0.65, 25.25) (0.5, -0.35, 27.25) (0.5, -0.35, 29.75) (0.5, -1.35, 31.75) (0.5, -1.35, 25.25) (0.5, -2.35, 27.25) (0.5, -2.35, 29.75) (0.5, -3.35, 31.75) (0.5, -3.35, 25.25) (0.5, -4.35, 27.25) (0.5, -4.35, 29.75) (0.5, -5.35, 31.75) (0.5, -5.35, 25.25) (0.5, -6.35, 27.25)
sketch "Sketch17" plane through (0.5, 0, 0) normal (1, 0, 0) x (0, 0, -1)
  point P0 (0, 0)
  point P1 (0, 16.3)
  point P2 (0, 11.7)
  point P3 (-1.626, 12.374)
  point P4 (-2.3, 14)
  point P5 (-1.626, 15.626)
  point P6 (2.3, 14)
  point P7 (1.626, 15.626)
  point P8 (1.626, 12.374)
  point P9 (0, -11.7)
  point P10 (0, -16.3)
  point P11 (-1.626, -15.626)
  point P12 (-2.3, -14)
  point P13 (-1.626, -12.374)
  point P14 (2.3, -14)
  point P15 (1.626, -12.374)
  point P16 (1.626, -15.626)
  constraints: 16 other
hole "Hole10" at (0.5, 16.3, 0) at (0.5, 11.7, 0) at (0.5, 12.374, 1.626) at (0.5, 14, 2.3) at (0.5, 15.626, 1.626) at (0.5, 14, -2.3) at (0.5, 15.626, -1.626) at (0.5, 12.374, -1.626) at (0.5, -11.7, 0) at (0.5, -16.3, 0) at (0.5, -15.626, 1.626) at (0.5, -14, 2.3) at (0.5, -12.374, 1.626) at (0.5, -14, -2.3) at (0.5, -12.374, -1.626) at (0.5, -15.626, -1.626) direction (-1, 0, 0) diameter 0.45 end through all
sketch "Sketch18" plane through (0.5, 0, 0) normal (1, 0, 0) x (0, 0, -1)
  point P0 (0, 0)
  point P1 (0, -7.55)
  constraints: 1 other
hole "Hole11" at (0.5, -7.55, 0) direction (-1, 0, 0) diameter 0.35 end through all
body "Solid2"
